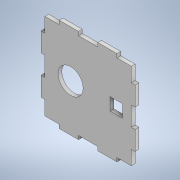
# Autodesk Inventor part: Bottom
Saved by Autodesk Inventor 2020 (Build 240168000, 168)
## iProperties
Created: 2020-12-28
Part Number: Bottom
Material: Generic
Document SubType Name: Modeling
Designer: solar
Density: 1 g/cm^3
Appearance: Default
Author: solar
Autodesk Inventor part; units mm, degrees
ref_plane "YZ Plane" through (0, 0, 0) normal (1, 0, 0) x (0, 1, 0)
ref_plane "XZ Plane" through (0, 0, 0) normal (0, 1, 0) x (-1, 0, 0)
ref_plane "XY Plane" through (0, 0, 0) normal (0, 0, 1) x (1, 0, 0)
sketch "Sketch1" plane through (0, 0, 0) normal (0, 0, 1) x (1, 0, 0)
  line L0 (-75, -15.375) -> (-69, -15.375)
  line L1 (-69, -46.125) -> (-75, -46.125)
  line L2 (-69, 46.125) -> (-75, 46.125)
  line L3 (-75, 15.375) -> (-69, 15.375)
  line L4 (-69, 46.125) -> (-69, 69)
  line L5 (-75, 46.125) -> (-75, 15.375)
  line L6 (-69, 15.375) -> (-69, -15.375)
  line L7 (-75, -15.375) -> (-75, -46.125)
  line L8 (-69, -46.125) -> (-69, -69)
  line L9 (0, 0) -> (0, 15.375)
  line L10 (0, 0) -> (0, -46.125)
  line L11 (69, 15.375) -> (69, -15.375)
  line L12 (75, 15.375) -> (69, 15.375)
  line L13 (75, 46.125) -> (75, 15.375)
  line L14 (69, 46.125) -> (75, 46.125)
  line L15 (69, 46.125) -> (69, 69)
  line L16 (75, -15.375) -> (69, -15.375)
  line L17 (75, -15.375) -> (75, -46.125)
  line L18 (69, -46.125) -> (75, -46.125)
  line L19 (69, -46.125) -> (69, -69)
  line L20 (0, 0) -> (92.4518, 92.4518)
  line L21 (0, 0) -> (130.7466, 0) construction
  line L22 (0, 0) -> (109.2471, 0) construction
  line L23 (0, 0) -> (102.0745, -102.0745)
  line L24 (0, 0) -> (162.0274, 0) construction
  line L25 (15.375, 69) -> (-15.375, 69)
  line L26 (15.375, 75) -> (15.375, 69)
  line L27 (46.125, 75) -> (15.375, 75)
  line L28 (46.125, 69) -> (46.125, 75)
  line L29 (46.125, 69) -> (69, 69)
  line L30 (-15.375, 75) -> (-15.375, 69)
  line L31 (-15.375, 75) -> (-46.125, 75)
  line L32 (-46.125, 69) -> (-46.125, 75)
  line L33 (-46.125, 69) -> (-69, 69)
  line L34 (-15.375, -75) -> (-15.375, -69)
  line L35 (-46.125, -69) -> (-46.125, -75)
  line L36 (46.125, -69) -> (46.125, -75)
  line L37 (15.375, -75) -> (15.375, -69)
  line L38 (46.125, -69) -> (69, -69)
  line L39 (46.125, -75) -> (15.375, -75)
  line L40 (15.375, -69) -> (-15.375, -69)
  line L41 (-15.375, -75) -> (-46.125, -75)
  line L42 (-46.125, -69) -> (-69, -69)
  line L43 (0, 0) -> (-28, 0)
  circle A0 centre (-28, 0) radius 20
  line L44 (0, 0) -> (45, 0)
  line L45 (35, 10) -> (55, 10)
  line L46 (55, 10) -> (55, -10)
  line L47 (55, -10) -> (35, -10)
  line L48 (35, -10) -> (35, 10)
  line L49 (35, 10) -> (55, -10) construction
  line L50 (55, 10) -> (35, -10) construction
  point P0 (0, 0)
  point P1 (-69, -75)
  point P2 (-69, 75)
  point P3 (69, -75)
  point P4 (69, 75)
  dimension "d8" = 45
  dimension "d13" = 28
  dimension "d14" = 40
  dimension "d15" = 45
  dimension "d16" = 20
  dimension "d17" = 20
  constraints: 102 end point, 18 symmetric about line, 5 point on line, 4 horizontal, 2 midpoint, 2 parallel, 2 perpendicular, 2 vertical, 1 centre point, 1 coincident, 1 equal length
  measures "d8" angle of L21 L20
  measures "d13" distance of L9.start L43.end
  measures "d14" diameter of A0
  measures "d15" distance of L9.start L44.end
  measures "d16" distance of L46.end L47.end
  measures "d17" distance of L45.end L46.end
extrude "Extrusion1" add sketch "Sketch1" along normal blind 6
body "Solid1"
